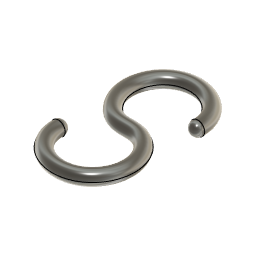
belt hook round v1 (Autodesk Fusion 360 design; units mm, degrees)
Autodesk Fusion 360 part; units mm, degrees
sketch "Sketch1" plane through (0, 0, 0) normal (0, 0, 1) x (1, 0, 0)
  line L0 (20, 30) -> (30, 30) construction
  line L1 (0, 30) -> (20, 30) construction
  arc A0 (20, 30) -> (0, 10) centre (0, 30) ccw
  arc A1 (30, 30) -> (-30, 29.9769) centre (0, 30) ccw
  line L2 (-20, -20) -> (-30, -20) construction
  arc A2 (-20, -20) -> (20, -20) centre (0, -20) ccw
  line L3 (0, -20) -> (-20, -20) construction
  arc A3 (-30, -20) -> (30, -19.9773) centre (0, -20) ccw
  spline S0 degree 5 poles (-30, 30) (-30, 27.543) (-29.6188, 22.8599) (-27.9033, 16.5274) (-23.6191, 9.5443) (-16.4104, 3.5431) (-8.9911, 0.4055) (-2.5301, -0.2698) (2.7256, 0.3103) (8.5619, -0.6894) (14.4606, -4.2613) (18.1587, -9.3307) (19.6651, -14.2542) (20, -18.0065) (20, -20) knots 0 0 0 0 0 0 0.1 0.2 0.3 0.4 0.5 0.6 0.7 0.8 0.9 1 1 1 1 1 1
  line L4 (20, -10) -> (20, -30)
  line L5 (-30, 40) -> (-30, 20)
  line L6 (-5, 0) -> (5, 0)
  spline S1 degree 5 poles (-20, 30) (-20, 29.9993) (-20, 29.9978) (-20, 29.9956) (-20, 29.9926) (-20, 29.9889) (-20, 29.986) (-20, 29.9838) (-20, 29.9823) (-20, 29.9815) knots 0 0 0 0 0 0 0.2 0.4 0.6 0.8 1 1 1 1 1 1
  line L7 (-20, 30.0019) -> (-20, 29.9981)
  line L8 (-20, 29.9834) -> (-20, 29.9797)
  spline S2 degree 5 poles (0, 10) (0.5503, 10) (2.2365, 10.0048) (5.1539, 9.9648) (9.7485, 9.2742) (16.4104, 6.4569) (23.6191, 0.4557) (27.9033, -6.5274) (29.6188, -12.8599) (30, -17.543) (30, -20) knots 0.451044 0.451044 0.451044 0.451044 0.451044 0.451044 0.5 0.6 0.7 0.8 0.9 1 1 1 1 1 1
  line L9 (-3.3857, 10) -> (3.3857, 10)
  line L10 (30, -12.5989) -> (30, -27.4011)
  line L11 (20, 30) -> (30, 30)
  line L12 (-30, -20) -> (-20, -20)
  spline S3 degree 5 poles (20, 30) (20, 29.7157) (20.0518, 29.1468) (20.2847, 28.2932) (20.8887, 27.1813) (22.0366, 25.983) (23.453, 25.1542) (25, 24.8507) (26.547, 25.1493) (27.9634, 25.9771) (29.1113, 27.1775) (29.7153, 28.2919) (29.9482, 29.1466) (30, 29.7157) (30, 30) knots 0 0 0 0 0 0 0.1 0.2 0.3 0.4 0.5 0.6 0.7 0.8 0.9 1 1 1 1 1 1
  line L13 (30, 29) -> (30, 31)
  line L14 (20, 31) -> (20, 29)
  line L15 (23.9196, 25.0016) -> (26.0804, 24.9984)
  spline S4 degree 5 poles (-30, -20) (-30, -19.7157) (-29.9489, -19.1467) (-29.7192, -18.2926) (-29.1222, -17.1794) (-27.9803, -15.98) (-26.5612, -15.1518) (-25, -14.8507) (-23.4388, -15.1518) (-22.0197, -15.98) (-20.8778, -17.1794) (-20.2808, -18.2926) (-20.0511, -19.1467) (-20, -19.7157) (-20, -20) knots 0 0 0 0 0 0 0.1 0.2 0.3 0.4 0.5 0.6 0.7 0.8 0.9 1 1 1 1 1 1
  line L16 (-20, -19) -> (-20, -21)
  line L17 (-30, -21) -> (-30, -19)
  arc A4 (-25, -15) -> (-25.0132, -15) centre (-25, -20) ccw
  arc A5 (-30, -20) -> (-30, -20) centre (-25, -20) ccw
  spline S5 degree 5 poles (-25, -20) (-25, -21.7234) (-24.7444, -25.057) (-23.5944, -29.718) (-20.5985, -35.2065) (-14.86, -40.5872) (-7.7497, -44.1527) (0.0158, -45.5851) (7.7158, -44.671) (14.699, -41.3839) (20.3917, -35.9012) (24.222, -28.5974) (25.7394, -20.0972) (24.2763, -11.1927) (19.8495, -3.1406) (13.5696, 2.5774) (6.5972, 5.2423) (0, 5) (-6.5972, 4.7577) (-13.5696, 7.4226) (-19.8495, 13.1406) (-24.2763, 21.1927) (-25.7394, 30.0972) (-24.222, 38.5974) (-20.3917, 45.9012) (-14.699, 51.3839) (-7.7158, 54.671) (-0.0158, 55.5851) (7.7497, 54.1527) (14.86, 50.5872) (20.5985, 45.2065) (23.5944, 39.718) (24.7444, 35.057) (25, 31.7234) (25, 30) knots 0 0 0 0 0 0 0.033333 0.066667 0.1 0.133333 0.166667 0.2 0.233333 0.266667 0.3 0.333333 0.366667 0.4 0.433333 0.466667 0.5 0.533333 0.566667 0.6 0.633333 0.666667 0.7 0.733333 0.766667 0.8 0.833333 0.866667 0.9 0.933333 0.966667 1 1 1 1 1 1
  line L18 (10, 5) -> (-10, 5)
  line L19 (-25, -7) -> (-25, -33)
  line L20 (25, -33) -> (25, -7)
  line L21 (-25, 17) -> (-25, 43)
  line L22 (25, 43) -> (25, 17)
  point P0 (0, 10)
  point P1 (25, 25)
  point P2 (0, -45)
  point P3 (25, -20)
  point P4 (0, 5)
  point P5 (-25, 30)
  point P6 (0, 55)
  constraint concentric A0 A1
  constraint horizontal L0
  constraint horizontal L1
  constraint coincident L1.start A0.centre
  constraint concentric A2 A3
  constraint coincident A2.centre L3.start
  constraint coincident A0 S1.start
  constraint coincident P0 A0.end
  constraint coincident A3 S2.end
  constraint coincident A1 S0.start
  constraint midpoint A2.end L4
  constraint midpoint S0.start L5
  constraint midpoint origin L6
  constraint coincident A0 S1.end
  constraint midpoint S1.start L7
  constraint midpoint S1.end L8
  constraint midpoint P0 L9
  constraint midpoint S2.end L10
  constraint coincident S0 A1.end
  constraint coincident S2 A3.end
  constraint midpoint L12 A4.centre
  constraint midpoint L0.end L13
  constraint midpoint L0.start L14
  constraint midpoint P1 L15
  constraint midpoint L2.start L16
  constraint tangent A2 L16
  constraint midpoint L2.end L17
  constraint coincident S4 A4.end
  constraint concentric A4 A5
  constraint coincident A4.centre A5.centre
  constraint midpoint L11 S5.end
  constraint midpoint P4 L18
  constraint midpoint A4.centre L19
  constraint midpoint P3 L20
  constraint midpoint P5 L21
  constraint midpoint S5.end L22
sketch "Sketch2" plane through (0, 0, 0) normal (0, 1, 0) x (1, 0, 0)
  circle A0 through (-20, 0, -20) (-27.5, 4.3301, -20) (-27.5, -4.3301, -20)
sweep "Sweep1" add profiles "Sketch2" path "Sketch1" along S5 section 1 contours A0 in plane through (0, -20, 0) normal (0, 1, 0)
sphere "SpherePrimitive1" add diameter 10 placed x (1, 0, 0) y (0, 0, 1) z (0, -1, 0) at (25, 30, 0)
sphere "SpherePrimitive2" add diameter 10 placed x (-1, 0, 0) y (0, 0, 1) z (0, 1, 0) at (-25, -20, 0)
